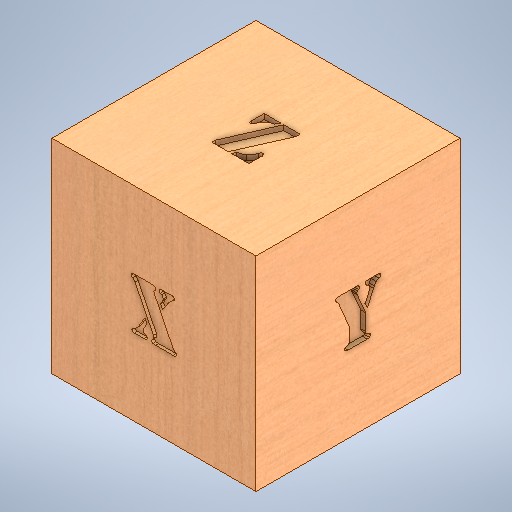
# Autodesk Inventor part: Sessao_2_0001_001
Saved by Autodesk Inventor 2025.2 (Build 292293000, 293)
## iProperties
Created: 2025-03-19
Part Number: Sessao_2_0001_001
Material: Wood (Cherry)
Document SubType Name: Modeling
Designer: ishad
Density: 0.63 g/cm^3
Appearance: Cherry - Natural Low Gloss
Author: ishad
Autodesk Inventor part; units mm, degrees
ref_plane "YZ Plane" through (0, 0, 0) normal (1, 0, 0) x (0, 1, 0)
ref_plane "XZ Plane" through (0, 0, 0) normal (0, 1, 0) x (-1, 0, 0)
ref_plane "XY Plane" through (0, 0, 0) normal (0, 0, 1) x (1, 0, 0)
sketch "Sketch1" plane through (0, 0, 0) normal (0, 0, 1) x (1, 0, 0)
  arc A0 (-31.0915, 14.1013) -> (-37.6725, 5.5506) centre (-29.9708, 6.4308) ccw
  line L0 (-31.0915, 14.1013) -> (-13.0692, 16.7345)
  arc A1 (-35.5154, -6.8969) -> (-33.1126, -2.4562) centre (-31.4973, -6.2006) ccw
  line L1 (-37.6725, 5.5506) -> (-35.5154, -6.8969)
  point P0 (0, 0)
  constraints: 4 end point, 4 point on circle, 2 centre point, 2 tangent
sketch "Sketch3" plane through (0, 0, 0) normal (0, 0, 1) x (1, 0, 0)
  line L0 (-25.1545, 0) -> (-37.9806, 19.4602)
  line L1 (26.1034, 1.4396) -> (37.7684, 19.1383)
  line L2 (0, 0) -> (0, 10)
  line L3 (-62.8603, 0) -> (-85.2801, 27.5944) construction
  line L4 (-62.8603, 0) -> (-112.8603, 0) construction
  line L5 (-96.3227, 24.2481) -> (-109.0709, 8.2649)
  dimension "d0" = 10
  dimension "d1" = 50
  dimension "d2" = 50.907
  constraints: 12 end point, 1 horizontal, 1 vertical, 1 other
  measures "d0" distance of L2.start L2.end
  measures "d1" distance of L3.start L4.end
  measures "d2" angle of L4 L3
sketch "Sketch4" plane through (0, 0, 0) normal (0, 0, 1) x (1, 0, 0)
  line L0 (-67.5733, 28.5005) -> (-17.5733, 28.5005)
  line L1 (7.4267, 78.5005) -> (7.4267, 28.5005)
  line L2 (-59.96, -30.5087) -> (-16.6675, -5.4934)
  line L3 (48.7587, -17.1375) -> (4.9787, 7.0143)
  line L4 (-17.5733, 28.5005) -> (7.4267, 28.5005)
  line L5 (-16.6675, -5.4934) -> (4.9787, 7.0143)
  line L6 (-96.3227, 24.2481) -> (-109.0709, 8.2649) projected
  line L7 (-62.8603, 0) -> (-85.2801, 27.5944) construction
  line L8 (-62.8603, 0) -> (-112.8603, 0) construction
  point P0 (0, 0)
  dimension "d3" = 50
  dimension "d4" = 25
  dimension "d5" = 50
  constraints: 12 end point, 4 equal length, 2 point on line, 1 horizontal
  measures "d3" distance of L0.start L0.end
  measures "d4" distance of L0.end L1.end
  measures "d5" distance of L1.start L1.end
sketch "Sketch5" plane through (0, 0, 0) normal (0, 0, 1) x (1, 0, 0)
  circle A0 centre (0, 0) radius 100
  circle A1 centre (0, 100) radius 15.6434
  circle A2 centre (-86.6025, 50) radius 15.6434
  circle A3 centre (-86.6025, -50) radius 15.6434
  circle A4 centre (0, -100) radius 15.6434
  circle A5 centre (86.6025, -50) radius 15.6434
  circle A6 centre (86.6025, 50) radius 15.6434
  circle A7 centre (-5.2336, 99.863) radius 15.6434
  circle A8 centre (-10.4528, 99.4522) radius 15.6434
  circle A9 centre (-15.6434, 98.7688) radius 15.6434
  circle A10 centre (-20.7912, 97.8148) radius 15.6434
  circle A11 centre (-25.8819, 96.5926) radius 15.6434
  circle A12 centre (-30.9017, 95.1057) radius 15.6434
  circle A13 centre (-35.8368, 93.358) radius 15.6434
  circle A14 centre (-40.6737, 91.3545) radius 15.6434
  circle A15 centre (-45.399, 89.1007) radius 15.6434
  circle A16 centre (-50, 86.6025) radius 15.6434
  circle A17 centre (-54.4639, 83.8671) radius 15.6434
  circle A18 centre (-58.7785, 80.9017) radius 15.6434
  circle A19 centre (-62.932, 77.7146) radius 15.6434
  circle A20 centre (-66.9131, 74.3145) radius 15.6434
  circle A21 centre (-70.7107, 70.7107) radius 15.6434
  circle A22 centre (-74.3145, 66.9131) radius 15.6434
  circle A23 centre (-77.7146, 62.932) radius 15.6434
  circle A24 centre (-80.9017, 58.7785) radius 15.6434
  circle A25 centre (-83.8671, 54.4639) radius 15.6434
  circle A26 centre (-86.6025, 50) radius 15.6434
  circle A27 centre (-89.1007, 45.399) radius 15.6434
  circle A28 centre (-91.3545, 40.6737) radius 15.6434
  circle A29 centre (-93.358, 35.8368) radius 15.6434
  circle A30 centre (-95.1057, 30.9017) radius 15.6434
  circle A31 centre (-96.5926, 25.8819) radius 15.6434
  circle A32 centre (-97.8148, 20.7912) radius 15.6434
  circle A33 centre (-98.7688, 15.6434) radius 15.6434
  circle A34 centre (-99.4522, 10.4528) radius 15.6434
  circle A35 centre (-99.863, 5.2336) radius 15.6434
  circle A36 centre (-100, 0) radius 15.6434
  circle A37 centre (-99.863, -5.2336) radius 15.6434
  circle A38 centre (-99.4522, -10.4528) radius 15.6434
  circle A39 centre (-98.7688, -15.6434) radius 15.6434
  circle A40 centre (-97.8148, -20.7912) radius 15.6434
  circle A41 centre (-96.5926, -25.8819) radius 15.6434
  circle A42 centre (-95.1057, -30.9017) radius 15.6434
  circle A43 centre (-93.358, -35.8368) radius 15.6434
  circle A44 centre (-91.3545, -40.6737) radius 15.6434
  circle A45 centre (-89.1007, -45.399) radius 15.6434
  circle A46 centre (-86.6025, -50) radius 15.6434
  circle A47 centre (-83.8671, -54.4639) radius 15.6434
  circle A48 centre (-80.9017, -58.7785) radius 15.6434
  circle A49 centre (-77.7146, -62.932) radius 15.6434
  circle A50 centre (-74.3145, -66.9131) radius 15.6434
  circle A51 centre (-70.7107, -70.7107) radius 15.6434
  circle A52 centre (-66.9131, -74.3145) radius 15.6434
  circle A53 centre (-62.932, -77.7146) radius 15.6434
  circle A54 centre (-58.7785, -80.9017) radius 15.6434
  circle A55 centre (-54.4639, -83.8671) radius 15.6434
  circle A56 centre (-50, -86.6025) radius 15.6434
  circle A57 centre (-45.399, -89.1007) radius 15.6434
  circle A58 centre (-40.6737, -91.3545) radius 15.6434
  circle A59 centre (-35.8368, -93.358) radius 15.6434
  circle A60 centre (-30.9017, -95.1057) radius 15.6434
  circle A61 centre (-25.8819, -96.5926) radius 15.6434
  circle A62 centre (-20.7912, -97.8148) radius 15.6434
  circle A63 centre (-15.6434, -98.7688) radius 15.6434
  circle A64 centre (-10.4528, -99.4522) radius 15.6434
  circle A65 centre (-5.2336, -99.863) radius 15.6434
  circle A66 centre (0, -100) radius 15.6434
  circle A67 centre (5.2336, -99.863) radius 15.6434
  circle A68 centre (10.4528, -99.4522) radius 15.6434
  circle A69 centre (15.6434, -98.7688) radius 15.6434
  circle A70 centre (20.7912, -97.8148) radius 15.6434
  circle A71 centre (25.8819, -96.5926) radius 15.6434
  circle A72 centre (30.9017, -95.1057) radius 15.6434
  circle A73 centre (35.8368, -93.358) radius 15.6434
  circle A74 centre (40.6737, -91.3545) radius 15.6434
  circle A75 centre (45.399, -89.1007) radius 15.6434
  circle A76 centre (50, -86.6025) radius 15.6434
  circle A77 centre (54.4639, -83.8671) radius 15.6434
  circle A78 centre (58.7785, -80.9017) radius 15.6434
  circle A79 centre (62.932, -77.7146) radius 15.6434
  circle A80 centre (66.9131, -74.3145) radius 15.6434
  circle A81 centre (70.7107, -70.7107) radius 15.6434
  circle A82 centre (74.3145, -66.9131) radius 15.6434
  circle A83 centre (77.7146, -62.932) radius 15.6434
  circle A84 centre (80.9017, -58.7785) radius 15.6434
  circle A85 centre (83.8671, -54.4639) radius 15.6434
  circle A86 centre (86.6025, -50) radius 15.6434
  circle A87 centre (89.1007, -45.399) radius 15.6434
  circle A88 centre (91.3545, -40.6737) radius 15.6434
  circle A89 centre (93.358, -35.8368) radius 15.6434
  circle A90 centre (95.1057, -30.9017) radius 15.6434
  circle A91 centre (96.5926, -25.8819) radius 15.6434
  circle A92 centre (97.8148, -20.7912) radius 15.6434
  circle A93 centre (98.7688, -15.6434) radius 15.6434
  circle A94 centre (99.4522, -10.4528) radius 15.6434
  circle A95 centre (99.863, -5.2336) radius 15.6434
  circle A96 centre (100, 0) radius 15.6434
  circle A97 centre (99.863, 5.2336) radius 15.6434
  circle A98 centre (99.4522, 10.4528) radius 15.6434
  circle A99 centre (98.7688, 15.6434) radius 15.6434
  circle A100 centre (97.8148, 20.7912) radius 15.6434
  circle A101 centre (96.5926, 25.8819) radius 15.6434
  circle A102 centre (95.1057, 30.9017) radius 15.6434
  circle A103 centre (93.358, 35.8368) radius 15.6434
  circle A104 centre (91.3545, 40.6737) radius 15.6434
  circle A105 centre (89.1007, 45.399) radius 15.6434
  circle A106 centre (86.6025, 50) radius 15.6434
  circle A107 centre (83.8671, 54.4639) radius 15.6434
  circle A108 centre (80.9017, 58.7785) radius 15.6434
  circle A109 centre (77.7146, 62.932) radius 15.6434
  circle A110 centre (74.3145, 66.9131) radius 15.6434
  circle A111 centre (70.7107, 70.7107) radius 15.6434
  circle A112 centre (66.9131, 74.3145) radius 15.6434
  circle A113 centre (62.932, 77.7146) radius 15.6434
  circle A114 centre (58.7785, 80.9017) radius 15.6434
  circle A115 centre (54.4639, 83.8671) radius 15.6434
  circle A116 centre (50, 86.6025) radius 15.6434
  circle A117 centre (45.399, 89.1007) radius 15.6434
  circle A118 centre (40.6737, 91.3545) radius 15.6434
  circle A119 centre (35.8368, 93.358) radius 15.6434
  circle A120 centre (30.9017, 95.1057) radius 15.6434
  circle A121 centre (25.8819, 96.5926) radius 15.6434
  circle A122 centre (20.7912, 97.8148) radius 15.6434
  circle A123 centre (15.6434, 98.7688) radius 15.6434
  circle A124 centre (10.4528, 99.4522) radius 15.6434
  circle A125 centre (5.2336, 99.863) radius 15.6434
  line L0 (0, 0) -> (100, 0) construction
  line L1 (0, 0) -> (0, 100) construction
  dimension "d6" = 200
  dimension "d9" = 360
  dimension "d13" = 360
  constraints: 125 centre point, 4 end point, 2 vertical alignment, 1 coincident, 1 horizontal, 1 tangent, 1 vertical, 256 other
sketch "Sketch6" plane through (0, 0, 0) normal (0, 0, 1) x (1, 0, 0)
  line L0 (0, 0) -> (0, 100.3698)
  line L1 (0, 0) -> (100.1353, 0)
  line L2 (10, 0) -> (10, 100.3698)
  line L3 (10, 0) -> (110.1353, 0)
  line L4 (0, 10) -> (0, 110.3698)
  line L5 (0, 10) -> (100.1353, 10)
  line L6 (10, 10) -> (10, 110.3698)
  line L7 (10, 10) -> (110.1353, 10)
  dimension "d17" = 10
  dimension "d20" = 10
  constraints: 16 end point, 2 collinear, 2 horizontal, 2 vertical, 13 other
  measures "d17" distance of L0.end L2.end
  measures "d20" distance of L0.end L4.end
sketch "Sketch7" plane through (0, 0, 0) normal (0, 0, 1) x (1, 0, 0)
  line L0 (100, -100) -> (-100, -100)
  line L1 (-100, -100) -> (-100, 100)
  line L2 (-100, 100) -> (100, 100)
  line L3 (100, 100) -> (100, -100)
  line L4 (100, -100) -> (-100, 100) construction
  line L5 (-100, -100) -> (100, 100) construction
  point P0 (0, 0)
  dimension "d23" = 200
  constraints: 12 end point, 2 midpoint, 2 parallel, 2 perpendicular, 1 horizontal
  measures "d23" distance of L1.end L2.end
extrude "Extrusion1" add sketch "Sketch7" along normal mid plane 200
sketch "Sketch8" plane through (0, 0, 100) normal (0, 0, 1) x (1, 0, 0)
  line L0 (-22.8082, 25) -> (22.8082, 25) construction
  line L1 (22.8082, 25) -> (22.8082, -25) construction
  line L2 (22.8082, -25) -> (-22.8082, -25) construction
  line L3 (-22.8082, -25) -> (-22.8082, 25) construction
  line L4 (-22.8082, 0) -> (0, 0)
  line L5 (0, 0) -> (22.8082, 0) construction
  line L6 (0.1519, 18.5764) -> (18.5981, -18.8802)
  spline S0 degree 2 poles (18.5981, -18.8802) (19.2491, -20.1823) (20.3776, -20.7465) knots 0 0 0 1 1 1
  spline S1 degree 2 poles (20.3776, -20.7465) (21.3759, -21.2674) (22.0703, -22.1354) (22.0703, -22.9167) knots 0 0 0 1 2 2 2
  spline S2 degree 2 poles (22.0703, -22.9167) (22.0703, -23.9149) (21.3325, -24.4792) knots 0 0 0 1 1 1
  spline S3 degree 2 poles (21.3325, -24.4792) (20.7248, -25) (18.6849, -25) knots 0 0 0 1 1 1
  line L7 (18.6849, -25) -> (1.4974, -25)
  spline S4 degree 2 poles (1.4974, -25) (-0.4557, -25) (-1.0634, -24.7396) knots 0 0 0 1 1 1
  spline S5 degree 2 poles (-1.0634, -24.7396) (-2.322, -24.1753) (-2.322, -22.8733) knots 0 0 0 1 1 1
  spline S6 degree 2 poles (-2.322, -22.8733) (-2.322, -22.3958) (-1.8012, -21.7014) (-1.1068, -21.1806) knots 0 0 0 1 2 2 2
  spline S7 degree 2 poles (-1.1068, -21.1806) (0.1085, -20.2691) (0.0651, -19.4878) knots 0 0 0 1 1 1
  spline S8 degree 2 poles (0.0651, -19.4878) (0.0217, -18.8802) (-0.5859, -17.6215) knots 0 0 0 1 1 1
  line L8 (-0.5859, -17.6215) -> (-18.5547, 18.5764)
  spline S9 degree 2 poles (-18.5547, 18.5764) (-18.9887, 19.4878) (-20.0304, 20.5729) (-20.855, 21.0069) knots 0 0 0 1 2 2 2
  spline S10 degree 2 poles (-20.855, 21.0069) (-21.5929, 21.3542) (-22.1571, 22.2656) (-22.1571, 23.0035) knots 0 0 0 1 2 2 2
  spline S11 degree 2 poles (-22.1571, 23.0035) (-22.1571, 24.1319) (-20.5946, 25) (-18.5547, 25) knots 0 0 0 1 2 2 2
  line L9 (-18.5547, 25) -> (-1.4974, 25)
  spline S12 degree 2 poles (-1.4974, 25) (0.3689, 25) (2.0182, 24.0451) (2.0182, 23.0035) knots 0 0 0 1 2 2 2
  spline S13 degree 2 poles (2.0182, 23.0035) (2.0182, 21.9184) (0.803, 21.1372) knots 0 0 0 1 1 1
  spline S14 degree 2 poles (0.803, 21.1372) (0.2387, 20.7031) (-0.1519, 20.1823) (-0.1519, 19.7049) knots 0 0 0 1 2 2 2
  spline S15 degree 2 poles (-0.1519, 19.7049) (-0.1519, 19.184) (0.1519, 18.5764) knots 0 0 0 1 1 1
  line L10 (-8.8759, -7.1181) -> (-6.8793, -11.2847)
  line L11 (-6.8793, -11.2847) -> (-9.1363, -15.0174)
  spline S16 degree 2 poles (-9.1363, -15.0174) (-10.395, -17.0573) (-10.395, -18.2726) knots 0 0 0 1 1 1
  spline S17 degree 2 poles (-10.395, -18.2726) (-10.395, -20.0087) (-8.4418, -20.8333) knots 0 0 0 1 1 1
  spline S18 degree 2 poles (-8.4418, -20.8333) (-7.3134, -21.2674) (-6.5321, -22.1354) (-6.5321, -22.9167) knots 0 0 0 1 2 2 2
  spline S19 degree 2 poles (-6.5321, -22.9167) (-6.5321, -23.9583) (-7.4002, -24.6094) knots 0 0 0 1 1 1
  spline S20 degree 2 poles (-7.4002, -24.6094) (-7.7474, -24.8698) (-8.5286, -25) (-9.6571, -25) knots 0 0 0 1 2 2 2
  line L12 (-9.6571, -25) -> (-19.1189, -25)
  spline S21 degree 2 poles (-19.1189, -25) (-20.2908, -25) (-21.6363, -24.0017) (-21.6363, -23.1337) knots 0 0 0 1 2 2 2
  spline S22 degree 2 poles (-21.6363, -23.1337) (-21.6363, -22.4392) (-20.8116, -21.5278) (-19.7266, -21.1372) knots 0 0 0 1 2 2 2
  spline S23 degree 2 poles (-19.7266, -21.1372) (-16.9922, -20.0521) (-15.4731, -17.6215) knots 0 0 0 1 1 1
  line L13 (-15.4731, -17.6215) -> (-8.8759, -7.1181)
  line L14 (8.3984, 8.4201) -> (6.3585, 12.5)
  line L15 (6.3585, 12.5) -> (8.3984, 15.9722)
  spline S24 degree 2 poles (8.3984, 15.9722) (9.0929, 17.1875) (9.0929, 18.0556) knots 0 0 0 1 1 1
  spline S25 degree 2 poles (9.0929, 18.0556) (9.0929, 18.8802) (8.0946, 20.3993) (7.3134, 20.7899) knots 0 0 0 1 2 2 2
  line L16 (7.3134, 20.7899) -> (6.0113, 21.3542)
  spline S26 degree 2 poles (6.0113, 21.3542) (5.6641, 21.5712) (5.0998, 22.5694) (5.0998, 23.0903) knots 0 0 0 1 2 2 2
  spline S27 degree 2 poles (5.0998, 23.0903) (5.0998, 23.9583) (6.3585, 25) (7.3568, 25) knots 0 0 0 1 2 2 2
  line L17 (7.3568, 25) -> (17.947, 25)
  spline S28 degree 2 poles (17.947, 25) (18.9887, 25) (20.3342, 24.0885) (20.3342, 23.3507) knots 0 0 0 1 2 2 2
  spline S29 degree 2 poles (20.3342, 23.3507) (20.3342, 22.4826) (19.6832, 21.8316) knots 0 0 0 1 1 1
  spline S30 degree 2 poles (19.6832, 21.8316) (19.4227, 21.5712) (18.1207, 20.8767) knots 0 0 0 1 1 1
  spline S31 degree 2 poles (18.1207, 20.8767) (15.5165, 19.4444) (13.8238, 16.7535) knots 0 0 0 1 1 1
  line L18 (13.8238, 16.7535) -> (8.3984, 8.4201)
  dimension "d26" = 50
  dimension "d27" = 45.6163
  constraints: 4 end point, 2 midpoint, 1 coincident, 1 horizontal, 2 other
  measures "d26" distance of L2.end L0.start
  measures "d27" distance of L0.start L0.end
extrude "Extrusion2" cut sketch "Sketch8" against normal blind 3
sketch "Sketch9" plane through (100, -100, 100) normal (1, 0, 0) x (0, 0, -1)
  line L0 (77.6042, 125) -> (122.3958, 125) construction
  line L1 (122.3958, 125) -> (122.3958, 75) construction
  line L2 (122.3958, 75) -> (77.6042, 75) construction
  line L3 (77.6042, 75) -> (77.6042, 125) construction
  line L4 (77.6042, 100) -> (100, 100) construction
  line L5 (100, 100) -> (122.3958, 100) construction
  line L6 (107.6823, 97.9167) -> (107.6823, 81.9444)
  spline S0 degree 2 poles (107.6823, 81.9444) (107.6823, 80.5122) (108.2465, 79.9045) knots 0 0 0 1 1 1
  spline S1 degree 2 poles (108.2465, 79.9045) (108.5069, 79.5573) (109.0278, 79.3403) (110.4601, 78.9931) knots 0 0 0 1 2 2 2
  spline S2 degree 2 poles (110.4601, 78.9931) (112.2396, 78.6024) (112.2396, 76.9965) knots 0 0 0 1 1 1
  spline S3 degree 2 poles (112.2396, 76.9965) (112.2396, 75.9115) (111.2413, 75.3472) knots 0 0 0 1 1 1
  spline S4 degree 2 poles (111.2413, 75.3472) (110.6771, 75) (108.9844, 75) knots 0 0 0 1 1 1
  line L7 (108.9844, 75) -> (107.7257, 75)
  line L8 (107.7257, 75) -> (91.3628, 75)
  line L9 (91.3628, 75) -> (90.1476, 75)
  spline S5 degree 2 poles (90.1476, 75) (88.4983, 75) (87.8472, 75.434) knots 0 0 0 1 1 1
  spline S6 degree 2 poles (87.8472, 75.434) (86.8924, 76.0417) (86.8924, 76.9965) knots 0 0 0 1 1 1
  spline S7 degree 2 poles (86.8924, 76.9965) (86.8924, 78.6024) (88.6719, 78.9931) knots 0 0 0 1 1 1
  spline S8 degree 2 poles (88.6719, 78.9931) (90.1042, 79.3403) (90.5816, 79.5573) (90.842, 79.9045) knots 0 0 0 1 2 2 2
  spline S9 degree 2 poles (90.842, 79.9045) (91.4062, 80.5122) (91.4062, 81.9444) knots 0 0 0 1 1 1
  line L10 (91.4062, 81.9444) -> (91.4062, 94.3142)
  line L11 (91.4062, 94.3142) -> (81.033, 119.0538)
  spline S10 degree 2 poles (81.033, 119.0538) (80.4687, 120.4427) (79.3837, 121.0938) knots 0 0 0 1 1 1
  spline S11 degree 2 poles (79.3837, 121.0938) (78.4288, 121.7014) (77.8646, 122.4392) (77.8646, 123.0903) knots 0 0 0 1 2 2 2
  spline S12 degree 2 poles (77.8646, 123.0903) (77.8646, 125) (80.6424, 125) knots 0 0 0 1 1 1
  line L12 (80.6424, 125) -> (98.6111, 125)
  spline S13 degree 2 poles (98.6111, 125) (100, 125) (100.5642, 124.6528) knots 0 0 0 1 1 1
  spline S14 degree 2 poles (100.5642, 124.6528) (101.4757, 124.0885) (101.4757, 123.1337) knots 0 0 0 1 1 1
  spline S15 degree 2 poles (101.4757, 123.1337) (101.4757, 121.9618) (100.434, 121.3108) knots 0 0 0 1 1 1
  line L13 (100.434, 121.3108) -> (99.349, 120.6597)
  spline S16 degree 2 poles (99.349, 120.6597) (98.7413, 120.2257) (98.7413, 119.4444) knots 0 0 0 1 1 1
  spline S17 degree 2 poles (98.7413, 119.4444) (98.7413, 118.533) (99.1319, 117.6215) knots 0 0 0 1 1 1
  line L14 (99.1319, 117.6215) -> (107.6823, 97.9167)
  line L15 (109.1146, 101.3889) -> (107.0312, 106.2066)
  line L16 (107.0312, 106.2066) -> (110.8941, 114.8003)
  spline S18 degree 2 poles (110.8941, 114.8003) (111.3715, 115.9288) (111.3715, 117.7951) knots 0 0 0 1 1 1
  spline S19 degree 2 poles (111.3715, 117.7951) (111.3715, 119.9219) (109.0278, 120.8767) knots 0 0 0 1 1 1
  spline S20 degree 2 poles (109.0278, 120.8767) (107.7691, 121.3542) (106.9878, 122.1354) (106.9878, 122.9601) knots 0 0 0 1 2 2 2
  spline S21 degree 2 poles (106.9878, 122.9601) (106.9878, 123.9583) (107.6389, 124.4358) knots 0 0 0 1 1 1
  spline S22 degree 2 poles (107.6389, 124.4358) (108.0729, 124.783) (109.158, 125) (110.5469, 125) knots 0 0 0 1 2 2 2
  line L17 (110.5469, 125) -> (119.5747, 125)
  spline S23 degree 2 poles (119.5747, 125) (122.1354, 125) (122.1354, 122.9601) knots 0 0 0 1 1 1
  spline S24 degree 2 poles (122.1354, 122.9601) (122.1354, 122.2222) (121.441, 121.3976) (120.4427, 120.9635) knots 0 0 0 1 2 2 2
  spline S25 degree 2 poles (120.4427, 120.9635) (118.6632, 120.1823) (117.8819, 119.3576) knots 0 0 0 1 1 1
  spline S26 degree 2 poles (117.8819, 119.3576) (116.7969, 118.1858) (116.059, 116.6667) knots 0 0 0 1 1 1
  line L18 (116.059, 116.6667) -> (115.2344, 114.8003)
  line L19 (115.2344, 114.8003) -> (109.1146, 101.3889)
  dimension "d30" = 44.7917
  dimension "d31" = 50
  constraints: 4 end point, 2 midpoint, 1 coincident, 1 horizontal, 2 other
  measures "d30" distance of L0.start L0.end
  measures "d31" distance of L2.end L0.start
extrude "Extrusion3" cut sketch "Sketch9" against normal blind 5
sketch "Sketch10" plane through (-100, 100, 100) normal (0, 1, 0) x (1, 0, 0)
  line L0 (80.3602, 125) -> (119.6398, 125) construction
  line L1 (119.6398, 125) -> (119.6398, 75) construction
  line L2 (119.6398, 75) -> (80.3602, 75) construction
  line L3 (80.3602, 75) -> (80.3602, 125) construction
  line L4 (80.3602, 100) -> (100, 100) construction
  line L5 (100, 100) -> (119.6398, 100) construction
  line L6 (118.1207, 125) -> (118.1207, 120.7899)
  line L7 (118.1207, 120.7899) -> (97.895, 75)
  line L8 (97.895, 75) -> (81.8793, 75)
  line L9 (81.8793, 75) -> (81.8793, 78.6458)
  line L10 (81.8793, 78.6458) -> (102.1918, 125)
  line L11 (102.1918, 125) -> (118.1207, 125)
  line L12 (118.1207, 75) -> (100.9766, 75)
  line L13 (100.9766, 75) -> (102.6259, 78.6458)
  spline S0 degree 2 poles (102.6259, 78.6458) (107.1398, 79.7309) (109.1363, 81.1198) knots 0 0 0 1 1 1
  spline S1 degree 2 poles (109.1363, 81.1198) (110.8724, 82.3351) (112.9991, 85.4601) (114.171, 88.6285) knots 0 0 0 1 2 2 2
  spline S2 degree 2 poles (114.171, 88.6285) (114.605, 89.8003) (115.4297, 90.625) (116.1675, 90.625) knots 0 0 0 1 2 2 2
  spline S3 degree 2 poles (116.1675, 90.625) (117.1224, 90.625) (118.1207, 89.3229) (118.1207, 88.0642) knots 0 0 0 1 2 2 2
  line L14 (118.1207, 88.0642) -> (118.1207, 75)
  line L15 (83.0946, 125) -> (98.98, 125)
  line L16 (98.98, 125) -> (97.1571, 120.8333)
  spline S4 degree 2 poles (97.1571, 120.8333) (94.0321, 120.3993) (91.428, 118.533) knots 0 0 0 1 1 1
  spline S5 degree 2 poles (91.428, 118.533) (88.1293, 116.2326) (86.9575, 111.8924) knots 0 0 0 1 1 1
  spline S6 degree 2 poles (86.9575, 111.8924) (86.6536, 110.7639) (85.7856, 109.8958) (84.9609, 109.8958) knots 0 0 0 1 2 2 2
  spline S7 degree 2 poles (84.9609, 109.8958) (83.0946, 109.8958) (83.0946, 112.0226) knots 0 0 0 1 1 1
  line L17 (83.0946, 112.0226) -> (83.0946, 125)
  point P0 (100, 100)
  dimension "d34" = 39.2795
  dimension "d35" = 50
  constraints: 4 end point, 2 midpoint, 1 coincident, 1 horizontal, 2 other
  measures "d34" distance of L0.start L0.end
  measures "d35" distance of L2.end L0.start
extrude "Extrusion4" cut sketch "Sketch10" against normal blind 5
equation "\"d24\" = d23"
body "Solid1"
